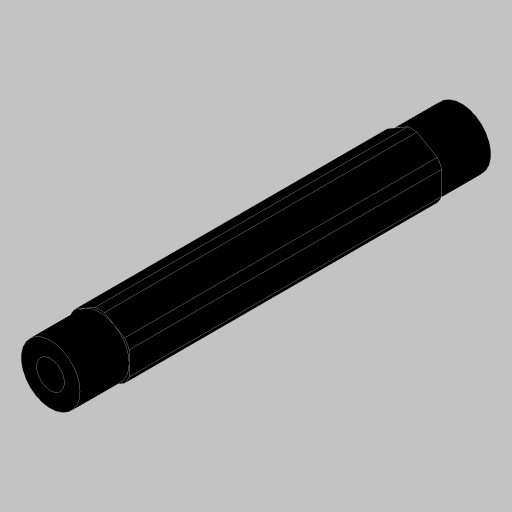
# Autodesk Inventor part: GP10-008
Saved by Autodesk Inventor 2023.5 (Build 275446000, 446)
## iProperties
RuleStatus: InUse
Created: 2025-03-09
Part Number: GP10-008
Material: Aluminum 6061
Document SubType Name: Modeling
Designer: brand
Mass: 8.50758 g
Surface Area: 25.7449 cm^2
Volume: 3.15096 cm^3
Density: 2.7 g/cm^3
Appearance: Anodized - Black
AfterDocNew0: SHOW
AfterDocOpen0: SHOW
AfterDocOpen1: size
AfterDocOpen2: thunder
BeforeDocSave0: size
BeforeDocSave1: thunder
AfterFeatureSuppressionChange0: thunder
AfterFeatureSuppressionChange1: size
PartBodyChanged0: thunder
PartBodyChanged1: size
AfterMaterialChange0: thunder
AfterMaterialChange1: size
Author: brand
Autodesk Inventor part; units mm, degrees
ref_plane "YZ Plane" through (0, 0, 0) normal (1, 0, 0) x (0, 1, 0)
ref_plane "XZ Plane" through (0, 0, 0) normal (0, 1, 0) x (-1, 0, 0)
ref_plane "XY Plane" through (0, 0, 0) normal (0, 0, 1) x (1, 0, 0)
sketch "Sketch1" plane through (0, 0, 0) normal (0, 0, 1) x (1, 0, 0)
  line L0 (-4.7625, -2.749631) -> (-4.7625, 2.749631)
  line L1 (-4.7625, 2.749631) -> (0, 5.499261)
  line L2 (0, 5.499261) -> (4.7625, 2.749631)
  line L3 (4.7625, 2.749631) -> (4.7625, -2.749631)
  line L4 (4.7625, -2.749631) -> (0, -5.499261)
  line L5 (0, -5.499261) -> (-4.7625, -2.749631)
  point P0 (0, 0)
  point P1 (0, 0)
  dimension "Size" = 9.525
  constraints: 12 end point, 1 coincident, 1 vertical alignment, 13 other
  measures "Size" distance between parallel lines of L3 L0
extrude "Extrusion1" add sketch "Sketch1" along normal mid plane 66.294
sketch "Sketch3" plane through (0, 0, 33.147) normal (0, 0, 1) x (1, 0, 0)
  line L0 (-4.7625, 2.749631) -> (0, 5.499261) construction
  line L1 (0, 5.499261) -> (4.7625, 2.749631) construction
  line L2 (4.7625, 2.749631) -> (4.7625, -2.749631) construction
  line L3 (4.7625, -2.749631) -> (0, -5.499261) construction
  line L4 (0, -5.499261) -> (-4.7625, -2.749631) construction
  line L5 (-4.7625, -2.749631) -> (-4.7625, 2.749631) construction
  point P0 (0, 0)
hole "Hole1" at (0, 0, 33.147) direction (0, 0, -1) diameter 4.4958 end through all
sketch "Sketch4" plane through (0, 0, 33.147) normal (0, 0, 1) x (1, 0, 0)
  circle A0 centre (0, 0) radius 2.2479 construction
  line L0 (-4.7625, 2.749631) -> (0, 5.499261) construction
  line L1 (0, 5.499261) -> (4.7625, 2.749631) construction
  line L2 (4.7625, 2.749631) -> (4.7625, -2.749631) construction
  line L3 (4.7625, -2.749631) -> (0, -5.499261) construction
  line L4 (0, -5.499261) -> (-4.7625, -2.749631) construction
  line L5 (-4.7625, -2.749631) -> (-4.7625, 2.749631) construction
  circle A1 centre (0, 0) radius 5.12445
  circle A2 centre (0, 0) radius 8.89
  dimension "thunder" = 10.2489
  dimension "d16" = 17.78
  constraints: 2 centre point, 2 coincident
  measures "thunder" diameter of A1
  measures "d16" diameter of A2
extrude "Extrusion3" cut sketch "Sketch4" against normal through all
sketch "Sketch5" plane through (0, 0, 33.147) normal (0, 0, 1) x (1, 0, 0)
  circle A0 centre (0, 0) radius 2.2479
  circle A1 centre (0, 0) radius 4.7625
  line L0 (4.7625, -1.891714) -> (4.7625, 1.891714)
  line L1 (4.019522, 3.178589) -> (0.742978, 5.070303)
  line L2 (-0.742978, 5.070303) -> (-4.019522, 3.178589)
  line L3 (-4.7625, 1.891714) -> (-4.7625, -1.891714)
  line L4 (-4.019522, -3.178589) -> (-0.742978, -5.070303)
  line L5 (0.742978, -5.070303) -> (4.019522, -3.178589)
  circle A2 centre (0, 0) radius 2.2479
  arc A3 (4.019522, -3.178589) -> (4.7625, -1.891714) centre (0, 0) ccw
  arc A4 (4.7625, 1.891714) -> (4.019522, 3.178589) centre (0, 0) ccw
  arc A5 (0.742978, 5.070303) -> (-0.742978, 5.070303) centre (0, 0) ccw
  arc A6 (-4.019522, 3.178589) -> (-4.7625, 1.891714) centre (0, 0) ccw
  arc A7 (-4.7625, -1.891714) -> (-4.019522, -3.178589) centre (0, 0) ccw
  arc A8 (-0.742978, -5.070303) -> (0.742978, -5.070303) centre (0, 0) ccw
  point P0 (2.38125, -4.124446)
  point P1 (-2.38125, -4.124446)
  point P2 (-4.7625, 0)
  point P3 (-2.38125, 4.124446)
  point P4 (2.38125, 4.124446)
  point P5 (4.7625, 0)
  dimension "d21" = 9.525
  constraints: 1 centre point, 1 coincident
  measures "d21" diameter of A1
extrude "Extrusion4" cut sketch "Sketch5" against normal blind 7.9248 contours L0 A3 L5 A1 | A1 L1 A4 L0 | A1 L2 A5 L1 | L5 A8 L4 A1 | A1 L3 A6 L2 | L4 A7 L3 A1
mirror "Mirror2" about plane through (0, 0, 0) normal (0, 0, 1) of "Extrusion4"
equation "\"bearing\" = 25.4"
body "Solid1"
